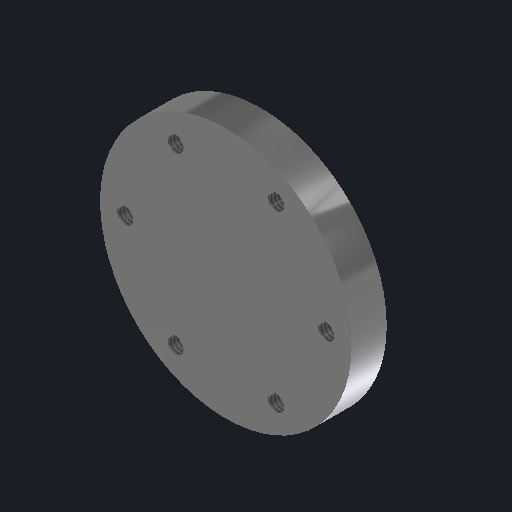
# Autodesk Inventor part: BridaTornillo
Saved by Autodesk Inventor 2022 (Build 260153000, 153)
## iProperties
Created: 2021-09-12
Part Number: BridaTornillo
Material: Stainless Steel, 440C
Document SubType Name: Modeling
Designer: Andres
Density: 7.75 g/cm^3
Appearance: Semi-Polished
Author: Andres
Autodesk Inventor part; units mm, degrees
ref_plane "YZ Plane" through (0, 0, 0) normal (1, 0, 0) x (0, 1, 0)
ref_plane "XZ Plane" through (0, 0, 0) normal (0, 1, 0) x (-1, 0, 0)
ref_plane "XY Plane" through (0, 0, 0) normal (0, 0, 1) x (1, 0, 0)
sketch "Sketch1" plane through (0, 0, 0) normal (0, 0, 1) x (1, 0, 0)
  arc A0 (6.5, 6.245) -> (6.5, -6.245) centre (1.5, 0) ccw projected
  line L0 (6.5, -6.245) -> (6.5, 6.245) projected
  circle A1 centre (1.5, 0) radius 8
  circle A2 centre (1.5, 0) radius 12
  point P0 (0, 0)
  point P1 (6.5, -6.245)
  point P2 (6.5, 6.245)
  dimension "d2" = 4
  constraints: 2 centre point, 2 coincident, 1 concentric
  measures "d2" radial gap between concentric circles of A2 A1
extrude "Extrusion1" add sketch "Sketch1" against normal blind 10
sketch "Sketch2" plane through (1.5, 0, 0) normal (0, 0, 1) x (1, 0, 0)
  circle A0 centre (0, 0) radius 12 projected
  circle A1 centre (0, 0) radius 8 projected
  circle A2 centre (0, 0) radius 25
  point P0 (-1.5, 0)
  dimension "d3" = 50
  constraints: 1 centre point, 1 coincident
  measures "d3" diameter of A2
extrude "Extrusion2" add sketch "Sketch2" along normal blind 2 and the other way blind 5 contours A0 | A1 | A2
chamfer "Chamfer1" distance 3 angle 45 1 edges at (-10.5, 0, -5)
ref_plane "Work Plane1" through (18.25, -40.5736, 0.0867) normal (1, 0, 0) x (0, 1, 0)
sketch "Sketch4" plane through (18.25, -40.5736, 0.0867) normal (1, 0, 0) x (0, 1, 0)
  line L0 (46.8186, -10.0867) -> (34.3286, -10.0867) projected
  line L1 (46.8186, -10.0867) -> (46.8186, -0.0867) projected
  line L2 (34.3286, -0.0867) -> (46.8186, -0.0867) projected
  line L3 (34.3286, -10.0867) -> (34.3286, -0.0867) projected
  line L4 (28.5736, -12.0867) -> (52.5736, -12.0867) projected
  point P0 (40.5736, -0.0867)
  point P1 (40.5736, -5.0867)
  point P2 (34.3286, -5.0867)
  point P3 (40.5736, -0.0867)
  point P4 (40.5736, -8.0867)
  point P5 (52.5736, -10.0867)
  point P6 (28.5736, -10.0867)
  point P7 (40.5736, -12.0867)
  dimension "d29" = 4
  constraints: 3 midpoint, 2 vertical alignment, 1 horizontal alignment
  measures "d29" distance from line of L4 point (40.574, -8.087)
hole "Hole2" at (18.25, 0, -8) direction (-1, 0, 0) diameter 2.459 depth 8.8 tip angle 118 thread size "M3x0.5" class "6H" standard "ISO Metric profile"
sketch "Sketch5" plane through (1.5, 0, 2) normal (0, 0, 1) x (1, 0, 0)
  circle A0 centre (0, 0) radius 25 projected
  circle A1 centre (0, 0) radius 20 construction
  point P0 (-1.5, 0)
  point P1 (-20, 0)
  point P2 (-10, -17.3205)
  point P3 (10, -17.3205)
  point P4 (20, 0)
  point P5 (10, 17.3205)
  point P6 (-10, 17.3205)
  dimension "d30" = 40
  dimension "d33" = 360
  constraints: 2 horizontal alignment, 1 coincident, 9 other
hole "Hole3" at (-18.5, 0, 2) at (-8.5, -17.3205, 2) at (11.5, -17.3205, 2) at (21.5, 0, 2) at (11.5, 17.3205, 2) at (-8.5, 17.3205, 2) direction (0, 0, -1) diameter 3.242 depth 6 tip angle 118 thread size "M4x0.7" class "6H" standard "ISO Metric profile"
body "Solid1"
